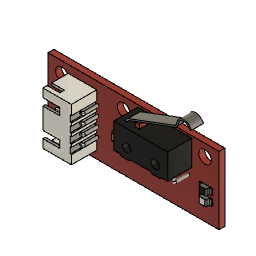
MetalFunk (Autodesk Fusion 360 archive; units mm, degrees)
design "End Stop Switch v5"
Autodesk Fusion 360 part; units mm, degrees
note: some values were not read from the file. Set by a fixed rule: which face or edge a step refers to.
sketch "Sketch1" plane through (0, 0, 0) normal (0, 1, 0) x (1, 0, 0)
  line L0 (20.25, 8.025) -> (-20.25, 8.025)
  line L1 (-20.25, 8.025) -> (-20.25, -8.025)
  line L2 (-20.25, -8.025) -> (20.25, -8.025)
  line L3 (20.25, -8.025) -> (20.25, 8.025)
  line L4 (20.25, 8.025) -> (-20.25, -8.025) construction
  line L5 (-20.25, 8.025) -> (20.25, -8.025) construction
  circle A0 centre (-16.95, -5.25) radius 1.5
  circle A1 centre (-16.95, 5.25) radius 1.5
  line L6 (-16.95, 5.25) -> (-16.95, -5.25) construction
  line L7 (-20.25, 0) -> (-16.95, 0) construction
  circle A2 centre (16.95, -5.25) radius 1.5
  line L8 (-16.95, -5.25) -> (16.95, -5.25) construction
  circle A3 centre (-2.35, -5.25) radius 1.5
  dimension "d1" = 40.5
  dimension "d2" = 16.05
  dimension "d3" = 3
  dimension "d4" = 10.5
  dimension "d5" = 3.3
  dimension "d6" = 3.3
  dimension "d7" = 3
  dimension "d8" = 14.6
  constraint horizontal L0
  constraint perpendicular L0 L1
  constraint parallel L0 L2
  constraint parallel L1 L3
  constraint coincident L4 origin
  constraint coincident L5 origin
  constraint equal A0 A1
  constraint coincident A1.centre L6.start
  constraint coincident A0.centre L6.end
  constraint vertical L6
  constraint midpoint L1 L7.start
  constraint midpoint L6 L7.end
  constraint horizontal L7
  constraint equal A0 A2
  constraint coincident A2.centre L8.end
  constraint horizontal L8
  constraint coincident L8 A3.centre
  measures "d1" distance of L0.start L0.end
  measures "d2" distance of L0.start L2.end
  measures "d3" diameter of A0
  measures "d4" distance of A0.centre A1.centre
  measures "d5" distance of L1 A0.centre
  measures "d6" distance of L3 A2.centre
  measures "d7" diameter of A3
  measures "d8" distance of A0.centre A3.centre
extrude "Extrude1" add sketch "Sketch1" along normal blind 1.4
sketch "Sketch2" plane through (0, 1.4, 0) normal (0, 1, 0) x (-1, 0, 0)
  circle A0 centre (2.35, 5.25) radius 1.5
  circle A1 centre (-16.95, 5.25) radius 1.5
  circle A2 centre (16.95, -5.25) radius 1.5
  circle A3 centre (16.95, 5.25) radius 1.5
  line L0 (-20.25, 8.025) -> (-20.25, -8.025)
  line L1 (-20.25, -8.025) -> (20.25, -8.025)
  line L2 (20.25, -8.025) -> (20.25, 8.025)
  line L3 (20.25, 8.025) -> (-20.25, 8.025)
  line L4 (7.75, 2.225) -> (9.25, 2.225)
  arc A4 (9.25, 2.225) -> (9.25, 4.025) centre (9.25, 3.125) ccw
  line L5 (9.25, 4.025) -> (7.75, 4.025)
  arc A5 (7.75, 4.025) -> (7.75, 2.225) centre (7.75, 3.125) ccw
  line L6 (7.75, 3.125) -> (9.25, 3.125) construction
  line L7 (9.25, 1.8583) -> (7.75, 1.8583)
  arc A6 (7.75, 1.8583) -> (7.75, 0.0583) centre (7.75, 0.9583) ccw
  line L8 (7.75, 0.0583) -> (9.25, 0.0583)
  arc A7 (9.25, 0.0583) -> (9.25, 1.8583) centre (9.25, 0.9583) ccw
  line L9 (9.25, -0.3083) -> (7.75, -0.3083)
  arc A8 (7.75, -0.3083) -> (7.75, -2.1083) centre (7.75, -1.2083) ccw
  line L10 (7.75, -2.1083) -> (9.25, -2.1083)
  arc A9 (9.25, -2.1083) -> (9.25, -0.3083) centre (9.25, -1.2083) ccw
  line L11 (9.25, -2.475) -> (7.75, -2.475)
  arc A10 (7.75, -2.475) -> (7.75, -4.275) centre (7.75, -3.375) ccw
  line L12 (7.75, -4.275) -> (9.25, -4.275)
  arc A11 (9.25, -4.275) -> (9.25, -2.475) centre (9.25, -3.375) ccw
  circle A12 centre (8.5, 3.125) radius 0.3
  circle A13 centre (8.5, 0.9583) radius 0.3
  circle A14 centre (8.5, -1.2083) radius 0.3
  circle A15 centre (8.5, -3.375) radius 0.3
  line L13 (-13.95, 0.475) -> (-13.95, -1.025)
  arc A16 (-13.95, -1.025) -> (-12.15, -1.025) centre (-13.05, -1.025) ccw
  line L14 (-12.15, -1.025) -> (-12.15, 0.475)
  arc A17 (-12.15, 0.475) -> (-13.95, 0.475) centre (-13.05, 0.475) ccw
  line L15 (-13.05, 0.475) -> (-13.05, -1.025) construction
  line L16 (-6.65, -1.025) -> (-6.65, 0.475)
  arc A18 (-6.65, 0.475) -> (-8.45, 0.475) centre (-7.55, 0.475) ccw
  line L17 (-8.45, 0.475) -> (-8.45, -1.025)
  arc A19 (-8.45, -1.025) -> (-6.65, -1.025) centre (-7.55, -1.025) ccw
  line L18 (-1.15, -1.025) -> (-1.15, 0.475)
  arc A20 (-1.15, 0.475) -> (-2.95, 0.475) centre (-2.05, 0.475) ccw
  line L19 (-2.95, 0.475) -> (-2.95, -1.025)
  arc A21 (-2.95, -1.025) -> (-1.15, -1.025) centre (-2.05, -1.025) ccw
  circle A22 centre (-13.05, -0.275) radius 0.3
  line L20 (-7.55, 0.475) -> (-7.55, -1.025) construction
  line L21 (-2.05, -1.025) -> (-2.05, 0.475) construction
  circle A23 centre (-7.55, -0.275) radius 0.3
  circle A24 centre (-2.05, -0.275) radius 0.3
  dimension "d11" = 1.8
  dimension "d12" = 1.5
  dimension "d13" = 4
  dimension "d14" = 11
  dimension "d17" = 0
  dimension "d18" = -6.5
  dimension "d19" = 0.6
  dimension "d30" = 1.5
  dimension "d31" = 1.8
  dimension "d32" = 7
  dimension "d33" = 7.2
  dimension "d36" = 11
  dimension "d37" = 0
  dimension "d38" = 0.6
  constraint tangent L4 A4
  constraint tangent A4 L5
  constraint parallel L4 L5
  constraint tangent L5 A5
  constraint tangent L4 A5
  constraint horizontal L6
  constraint midpoint L6 A12.centre
  constraint equal A14 A15
  constraint equal A13 A14
  constraint equal A12 A13
  constraint tangent L13 A16
  constraint tangent A16 L14
  constraint parallel L13 L14
  constraint tangent L14 A17
  constraint tangent L13 A17
  constraint parallel L0 L15
  constraint midpoint L15 A22.centre
  constraint coincident A18.centre L20.start
  constraint coincident A19.centre L20.end
  constraint coincident A21.centre L21.start
  constraint coincident A20.centre L21.end
  constraint midpoint L20 A23.centre
  constraint midpoint L21 A24.centre
  constraint equal A22 A23
  constraint equal A23 A24
  measures "d11" distance of L4 L5
  measures "d12" distance of A5.centre A4.centre
  measures "d13" distance of L3 L5
  measures "d14" distance of L2 A4.centre
  measures "d19" diameter of A15
  measures "d30" distance of A17.centre A16.centre
  measures "d31" distance of L13 L14
  measures "d32" distance of L1 A16.centre
  measures "d33" distance of L0 A16.centre
  measures "d38" diameter of A22
extrude "Extrude6" add sketch "Sketch2" against normal blind 4.35 contours A12 | A13 | A14 | A15
extrude "Extrude2" add sketch "Sketch2" along normal blind 0.5 contours L4 A4 L5 A5 | L7 A6 L8 A7 | L9 A8 L10 A9 | L11 A10 L12 A11 | L13 A16 L14 A17 | L16 A18 L17 A19 | L18 A20 L19 A21
extrude "Extrude3" add sketch "Sketch2" along normal blind 2 contours A12 | A13 | A14 | A15 | A22 | A23 | A24
fillet "Fillet1" radius 0.3 1 faces at (-8.4925, 1.9, -4.0747)
fillet "Fillet2" radius 0.3 3 faces at (-8.4925, 1.9, -1.9081) (-8.4925, 1.9, 0.2586) (-8.4925, 1.9, 2.4253)
fillet "Fillet2" radius 0.3 3 faces at (13.75, 1.9, -0.275) (6.85, 1.9, -0.275) (2.75, 1.9, -0.275)
fillet "Fillet3" radius 0.1 1 edges at (-8.2203, 3.4, 3.0165) 4 faces at (-8.4377, 3.4, -3.5121) (-8.4377, 3.4, -1.3455) (-8.4267, 3.4, 0.8314) (-8.4377, 3.4, 2.9879)
fillet "Fillet3" radius 0.1 3 faces at (2.1033, 3.4, -0.0705) (7.6233, 3.4, -0.148) (12.9767, 3.4, -0.148)
sketch "Sketch3" plane through (0, 0, 0) normal (0, -1, 0) x (1, 0, 0)
  circle A0 centre (-2.35, 5.25) radius 1.5
  circle A1 centre (16.95, 5.25) radius 1.5
  circle A2 centre (-16.95, -5.25) radius 1.5
  circle A3 centre (-16.95, 5.25) radius 1.5
  line L0 (20.25, -8.025) -> (20.25, 8.025)
  line L1 (20.25, 8.025) -> (-20.25, 8.025)
  line L2 (-20.25, 8.025) -> (-20.25, -8.025)
  line L3 (-20.25, -8.025) -> (20.25, -8.025)
  line L4 (-15.45, 6.2) -> (-8.7, 6.2)
  line L5 (-8.7, 6.2) -> (-8.7, -6.2)
  line L6 (-8.7, -6.2) -> (-15.45, -6.2)
  line L7 (-15.45, -6.2) -> (-15.45, 6.2)
  line L8 (-20.25, 0) -> (-15.45, 0) construction
  circle A4 centre (-8.5, -3.375) radius 0.3
  circle A5 centre (-8.5, 0.9583) radius 0.3
  circle A6 centre (-8.5, -1.2083) radius 0.3
  circle A7 centre (-8.5, 3.125) radius 0.3
  dimension "d43" = 12.4
  dimension "d44" = 6.75
  constraint horizontal L4
  constraint vertical L5
  constraint horizontal L6
  constraint vertical L7
  constraint tangent A3 L7
  constraint midpoint L2 L8.start
  constraint midpoint L7 L8.end
  constraint horizontal L8
  measures "d43" distance of L4 L6
  measures "d44" distance of L4.start L4.end
extrude "Extrude4" add sketch "Sketch3" along normal blind 6 contours L4 L5 L6 L7 A4 A5 A6 A7 | L5 A4 | L5 A7 | L5 A6 | L5 A5 picked at (-8.7489, -3.4027) picked at (-8.7504, 3.1324) picked at (-8.718, -1.2615) picked at (-8.7504, 0.9657)
sketch "Sketch4" plane through (-15.45, 0, 0) normal (-1, 0, 0) x (0, -1, 0)
  line L0 (0, -5.25) -> (0, -6.2)
  line L1 (0, -6.2) -> (6, -6.2)
  line L2 (6, -6.2) -> (6, 6.2)
  line L3 (6, 6.2) -> (0, 6.2)
  line L4 (0, 6.2) -> (0, 5.25)
  line L5 (0, 5.25) -> (0, -5.25)
  line L6 (0.6, 5.6) -> (0.6, 5.25)
  line L7 (0.6, 5.25) -> (0.6, -5.25)
  line L8 (0.6, -5.25) -> (0.6, -5.6)
  line L9 (0.6, -5.6) -> (5.4, -5.6)
  line L10 (5.4, -5.6) -> (5.4, 5.6)
  line L11 (5.4, 5.6) -> (0.6, 5.6)
  dimension "d47" = -0.6
extrude "Extrude5" cut sketch "Sketch4" against normal blind 6.15 contours L6 L7 L8 L9 L10 L11
ref_plane "WorkPlane1" through (-12.075, -3, 3.2) normal (0, 0, 1) x (-1, 0, 0)
sketch "Sketch6" plane through (0, -6, 0) normal (0, -1, 0) x (1, 0, 0)
  line L0 (-15.45, -6.2) -> (-8.7, -6.2)
  line L1 (-8.7, 1.7083) -> (-8.7, 2.375)
  line L2 (-8.7, 6.2) -> (-15.45, 6.2)
  line L3 (-15.45, 6.2) -> (-15.45, -6.2)
  line L4 (-15.45, 4.2) -> (-11.45, 4.2)
  line L5 (-11.45, 4.2) -> (-11.45, 2.5)
  line L6 (-11.45, 2.5) -> (-15.45, 2.5)
  line L7 (-15.45, 2.5) -> (-15.45, 4.2)
  line L8 (-15.45, -2.5) -> (-11.45, -2.5)
  line L9 (-11.45, -2.5) -> (-11.45, -4.2)
  line L10 (-11.45, -4.2) -> (-15.45, -4.2)
  line L11 (-15.45, -4.2) -> (-15.45, -2.5)
  line L12 (-9, 1.7083) -> (-8.7, 1.7083)
  line L13 (-8.7, 2.375) -> (-9, 2.375)
  line L14 (-9, 2.375) -> (-9, 3.875)
  line L15 (-9, 3.875) -> (-8.7, 3.875)
  line L16 (-8.7, 3.875) -> (-8.7, 6.2)
  line L17 (-8.7, -6.2) -> (-8.7, -4.125)
  line L18 (-8.7, -4.125) -> (-9, -4.125)
  line L19 (-9, -4.125) -> (-9, -2.625)
  line L20 (-9, -2.625) -> (-8.7, -2.625)
  line L21 (-8.7, -2.625) -> (-8.7, -1.9583)
  line L22 (-8.7, -1.9583) -> (-9, -1.9583)
  line L23 (-9, -1.9583) -> (-9, -0.4583)
  line L24 (-9, -0.4583) -> (-8.7, -0.4583)
  line L25 (-8.7, -0.4583) -> (-8.7, 0.2083)
  line L26 (-8.7, 0.2083) -> (-9, 0.2083)
  line L27 (-9, 0.2083) -> (-9, 1.7083)
  dimension "d62" = 1.7
  dimension "d63" = 1.7
  dimension "d64" = 4
  dimension "d65" = 4
  dimension "d66" = 2
  dimension "d67" = 2
  constraint horizontal L4
  constraint vertical L5
  constraint horizontal L6
  constraint vertical L7
  constraint coincident L3 L4.start
  constraint horizontal L8
  constraint vertical L9
  constraint horizontal L10
  constraint vertical L11
  constraint coincident L3 L8.start
  measures "d62" distance of L4 L6
  measures "d63" distance of L8 L10
  measures "d64" distance of L5.end L6.end
  measures "d65" distance of L9.end L10.end
  measures "d66" distance of L2 L4
  measures "d67" distance of L0 L10
extrude "Extrude8" cut sketch "Sketch6" against normal blind 1 contours L3 L8 L9 L10 L11 | L3 L4 L5 L6 L7
sketch "Sketch5" plane through (-12.075, -3, 3.2) normal (0, 0, 1) x (1, 0, 0)
  line L0 (3.6, 0.05) -> (3.6, -0.2)
  line L1 (3.3, -0.5) -> (2.75, -0.5)
  arc A0 (3.3, -0.5) -> (3.6, -0.2) centre (3.3, -0.2) ccw
  dimension "d53" = 0.3
  constraint vertical L0
  constraint perpendicular L0 L1
  constraint tangent L1 A0
  constraint tangent L0 A0
  measures "d53" radius of A0
sweep "Sweep1" add 4 faces at (-8.5336, -2.95, 3.1176) (-8.5336, -2.95, 0.9509) (-8.5336, -2.95, -1.2157) (-8.5336, -2.95, -3.3824) path "Sketch5" along L1 A0 L0
sketch "Sketch7" plane through (0, -6, 0) normal (0, -1, 0) x (1, 0, 0)
  line L0 (-11.45, 2.5) -> (-15.45, 2.5)
  line L1 (-15.45, 2.5) -> (-15.45, -2.5)
  line L2 (-15.45, -2.5) -> (-11.45, -2.5)
  line L3 (-11.45, -2.5) -> (-11.45, -4.2)
  line L4 (-11.45, -4.2) -> (-15.45, -4.2)
  line L5 (-15.45, -4.2) -> (-15.45, -6.2)
  line L6 (-15.45, -6.2) -> (-8.7, -6.2)
  line L7 (-8.7, -6.2) -> (-8.7, 6.2)
  line L8 (-8.7, 6.2) -> (-15.45, 6.2)
  line L9 (-15.45, 6.2) -> (-15.45, 4.2)
  line L10 (-15.45, 4.2) -> (-11.45, 4.2)
  line L11 (-11.45, 4.2) -> (-11.45, 2.5)
  line L12 (-8.7, 3.875) -> (-9, 3.875)
  line L13 (-9, 3.875) -> (-9, 2.375)
  line L14 (-9, 2.375) -> (-8.7, 2.375)
  line L15 (-8.7, 2.375) -> (-8.7, 3.875)
  arc A0 (-8.7, 2.9014) -> (-8.7, 3.3486) centre (-8.5, 3.125) ccw construction
  line L16 (-9, 3.125) -> (-8.5, 3.125) construction
  line L17 (-8.7, 1.7083) -> (-9, 1.7083)
  line L18 (-8.7, 0.2083) -> (-8.7, 1.7083)
  line L19 (-9, 1.7083) -> (-9, 0.2083)
  line L20 (-9, 0.2083) -> (-8.7, 0.2083)
  line L21 (-8.7, -0.4583) -> (-9, -0.4583)
  line L22 (-8.7, -1.9583) -> (-8.7, -0.4583)
  line L23 (-9, -0.4583) -> (-9, -1.9583)
  line L24 (-9, -1.9583) -> (-8.7, -1.9583)
  line L25 (-8.7, -2.625) -> (-9, -2.625)
  line L26 (-8.7, -4.125) -> (-8.7, -2.625)
  line L27 (-9, -2.625) -> (-9, -4.125)
  line L28 (-9, -4.125) -> (-8.7, -4.125)
  dimension "d70" = 0.3
  dimension "d71" = 1.5
  dimension "d74" = 0
  dimension "d75" = -6.5
  constraint horizontal L12
  constraint vertical L13
  constraint horizontal L14
  constraint vertical L15
  constraint coincident L7 L12.start
  constraint midpoint L13 L16.start
  constraint coincident A0.centre L16.end
  constraint horizontal L16
  measures "d70" distance of L13.end L14.end
  measures "d71" distance of L12.end L13.end
extrude "Extrude9" cut sketch "Sketch7" against normal blind 6 contours L7 L12 L13 L14 L15 | L7 L17 L18 L19 L20 | L7 L25 L26 L27 L28 | L7 L21 L22 L23 L24
extrude "Extrude7" add 4 faces at (-9.325, -3.4102, 3.0521) (-9.325, -3.4102, 0.8855) (-9.325, -3.4102, -1.2812) (-9.325, -3.4102, -3.4479) along direction (-1, 0, 0) blind 5.5 and the other way blind 0.63
sketch "Sketch8" plane through (0, 0, -6.2) normal (0, 0, -1) x (1, 0, 0)
  line L0 (-15.45, 0) -> (-8.7, 0)
  line L1 (-8.7, 0) -> (-8.7, 6)
  line L2 (-8.7, 6) -> (-15.45, 6)
  line L3 (-15.45, 6) -> (-15.45, 0)
  line L4 (-15.45, 5) -> (-12.45, 5)
  line L5 (-12.45, 5) -> (-12.45, 3.9)
  line L6 (-12.45, 3.9) -> (-15.45, 3.9)
  line L7 (-15.45, 3.9) -> (-15.45, 5)
  dimension "d80" = 1.1
  dimension "d81" = 1
  dimension "d82" = 3
  constraint horizontal L4
  constraint vertical L5
  constraint horizontal L6
  constraint vertical L7
  constraint coincident L3 L4.start
  measures "d80" distance of L4.end L5.end
  measures "d81" distance of L2 L4
  measures "d82" distance of L5.end L6.end
extrude "Extrude10" cut sketch "Sketch8" against normal blind 1 contours L3 L4 L5 L6 L7
mirror "Mirror1" about plane through (0, 0, 0) normal (0, 0, 1) of "Extrude10"
sketch "Sketch9" plane through (0, 0, 0) normal (0, -1, 0) x (1, 0, 0)
  arc A0 (-8.7, 0.7347) -> (-8.7, 1.1819) centre (-8.5, 0.9583) ccw
  line L0 (-8.7, 0.7347) -> (-8.7, 1.1819)
  arc A1 (-8.7, -1.4319) -> (-8.7, -0.9847) centre (-8.5, -1.2083) ccw
  line L1 (-8.7, -1.4319) -> (-8.7, -0.9847)
  arc A2 (-8.7, 2.9014) -> (-8.7, 3.3486) centre (-8.5, 3.125) ccw
  line L2 (-8.7, 2.9014) -> (-8.7, 3.3486)
  line L3 (-8.7, 1.7083) -> (-9, 1.7083)
  line L4 (-9, 1.7083) -> (-9, 0.2083)
  line L5 (-9, 0.2083) -> (-8.7, 0.2083)
  line L6 (-8.7, 0.2083) -> (-8.7, -0.4583)
  line L7 (-8.7, -0.4583) -> (-9, -0.4583)
  line L8 (-9, -0.4583) -> (-9, -1.9583)
  line L9 (-9, -1.9583) -> (-8.7, -1.9583)
  line L10 (-8.7, -1.9583) -> (-8.7, -2.625)
  line L11 (-8.7, -2.625) -> (-9, -2.625)
  line L12 (-9, -2.625) -> (-9, -4.125)
  line L13 (-9, -4.125) -> (-8.7, -4.125)
  line L14 (-8.7, -4.125) -> (-8.7, -6.2)
  line L15 (-8.7, -6.2) -> (-15.45, -6.2)
  line L16 (-15.45, -6.2) -> (-15.45, -5.25)
  circle A3 centre (-16.95, -5.25) radius 1.5
  line L17 (-15.45, -5.25) -> (-15.45, 5.25)
  circle A4 centre (-16.95, 5.25) radius 1.5
  line L18 (-15.45, 5.25) -> (-15.45, 6.2)
  line L19 (-15.45, 6.2) -> (-8.7, 6.2)
  line L20 (-8.7, 6.2) -> (-8.7, 3.875)
  line L21 (-8.7, 3.875) -> (-9, 3.875)
  line L22 (-9, 3.875) -> (-9, 2.375)
  line L23 (-9, 2.375) -> (-8.7, 2.375)
  line L24 (-8.7, 2.375) -> (-8.7, 1.7083)
  line L25 (20.25, -8.025) -> (20.25, 8.025)
  line L26 (20.25, 8.025) -> (-20.25, 8.025)
  line L27 (-20.25, 8.025) -> (-20.25, -8.025)
  line L28 (-20.25, -8.025) -> (20.25, -8.025)
  circle A5 centre (16.95, 5.25) radius 1.5
  circle A6 centre (-2.35, 5.25) radius 1.5
  line L29 (-8.7, -3.5986) -> (-8.7, -3.1514)
  arc A7 (-8.7, -3.5986) -> (-8.7, -3.1514) centre (-8.5, -3.375) ccw
  line L30 (-4.15, 0.475) -> (-2.75, 0.475)
  line L31 (-2.75, 0.475) -> (-2.75, -1.725)
  line L32 (-2.75, -1.725) -> (-4.15, -1.725)
  line L33 (-4.15, -1.725) -> (-4.15, 0.475)
  line L34 (-4.15, 0.875) -> (-2.75, 0.875)
  line L35 (-2.75, 0.875) -> (-2.75, -2.125)
  line L36 (-2.75, -2.125) -> (-4.15, -2.125)
  line L37 (-4.15, -2.125) -> (-4.15, 0.875)
  line L38 (-4.15, -0.625) -> (-2.75, -0.625) construction
  line L39 (-0.05, 0.875) -> (-0.0503, 0.8857)
  line L40 (-1.95, 0.8566) -> (-1.95, 0.875)
  line L41 (-1.95, 0.875) -> (-0.55, 0.875)
  line L42 (-0.55, 0.875) -> (-0.55, -2.125)
  line L43 (-0.55, -2.125) -> (-1.95, -2.125)
  line L44 (-1.95, -2.125) -> (-1.95, 0.875)
  line L45 (-1.95, 0.475) -> (-0.55, 0.475)
  line L46 (-0.55, 0.475) -> (-0.55, -1.725)
  line L47 (-0.55, -1.725) -> (-1.95, -1.725)
  line L48 (-1.95, -1.725) -> (-1.95, 0.475)
  dimension "d87" = 2.2
  dimension "d88" = 1.4
  dimension "d89" = 8.5
  dimension "d90" = 17.5
  dimension "d91" = 3
  dimension "d97" = 0.8
  constraint horizontal L30
  constraint vertical L31
  constraint horizontal L32
  constraint vertical L33
  constraint horizontal L34
  constraint vertical L35
  constraint horizontal L36
  constraint vertical L37
  constraint collinear L33 L37
  constraint collinear L31 L35
  constraint midpoint L37 L38.start
  constraint midpoint L35 L38.end
  constraint symmetric L30 L32 L38
  constraint horizontal L41
  constraint vertical L42
  constraint horizontal L43
  constraint vertical L44
  constraint equal L36 L43
  constraint equal L37 L44
  constraint horizontal L45
  constraint vertical L46
  constraint horizontal L47
  constraint vertical L48
  constraint coincident L42 L46.end
  constraint coincident L44 L45.start
  constraint collinear L32 L47
  constraint collinear L30 L45
  constraint collinear L34 L41
  measures "d87" distance of L30.end L31.end
  measures "d88" distance of L31.end L32.end
  measures "d89" distance of L28 L30
  measures "d90" distance of L27 L31
  measures "d91" distance of L34 L36
  measures "d97" distance of L35 L40
extrude "Extrude11" add sketch "Sketch9" along normal blind 0.2 contours L30 L34 L35 L37 | L32 L35 L36 L37 | L40 L41 L42 L44 L45 | L42 L43 L44 L47
extrude "Extrude12" add sketch "Sketch9" along normal blind 1 contours L30 L31 L32 L33 L35 L37 | L42 L44 L45 L46 L47 L48
fillet "Fillet4" radius 0.4 4 edges at (-3.45, -1, -1.725) (-3.45, -1, 0.475) (-1.25, -1, 0.475) (-1.25, -1, -1.725)
sketch "Sketch10" plane through (0, 0, 0) normal (0, -1, 0) x (1, 0, 0)
  line L0 (-0.55, 0.875) -> (-0.55, -2.125)
  line L1 (-0.55, -2.125) -> (-1.95, -2.125)
  line L2 (-1.95, -2.125) -> (-1.95, 0.875)
  line L3 (-1.95, 0.875) -> (-0.55, 0.875)
  line L4 (-8.7, -3.5986) -> (-8.7, -3.1514)
  arc A0 (-8.7, -3.5986) -> (-8.7, -3.1514) centre (-8.5, -3.375) ccw
  circle A1 centre (-2.35, 5.25) radius 1.5
  circle A2 centre (16.95, 5.25) radius 1.5
  line L5 (20.25, -8.025) -> (20.25, 8.025)
  line L6 (20.25, 8.025) -> (-20.25, 8.025)
  line L7 (-20.25, 8.025) -> (-20.25, -8.025)
  line L8 (-20.25, -8.025) -> (20.25, -8.025)
  line L9 (-8.7, 1.7083) -> (-9, 1.7083)
  line L10 (-9, 1.7083) -> (-9, 0.2083)
  line L11 (-9, 0.2083) -> (-8.7, 0.2083)
  line L12 (-8.7, 0.2083) -> (-8.7, -0.4583)
  line L13 (-8.7, -0.4583) -> (-9, -0.4583)
  line L14 (-9, -0.4583) -> (-9, -1.9583)
  line L15 (-9, -1.9583) -> (-8.7, -1.9583)
  line L16 (-8.7, -1.9583) -> (-8.7, -2.625)
  line L17 (-8.7, -2.625) -> (-9, -2.625)
  line L18 (-9, -2.625) -> (-9, -4.125)
  line L19 (-9, -4.125) -> (-8.7, -4.125)
  line L20 (-8.7, -4.125) -> (-8.7, -6.2)
  line L21 (-8.7, -6.2) -> (-15.45, -6.2)
  line L22 (-15.45, -6.2) -> (-15.45, -5.25)
  circle A3 centre (-16.95, -5.25) radius 1.5
  line L23 (-15.45, -5.25) -> (-15.45, 5.25)
  circle A4 centre (-16.95, 5.25) radius 1.5
  line L24 (-15.45, 5.25) -> (-15.45, 6.2)
  line L25 (-15.45, 6.2) -> (-8.7, 6.2)
  line L26 (-8.7, 6.2) -> (-8.7, 3.875)
  line L27 (-8.7, 3.875) -> (-9, 3.875)
  line L28 (-9, 3.875) -> (-9, 2.375)
  line L29 (-9, 2.375) -> (-8.7, 2.375)
  line L30 (-8.7, 2.375) -> (-8.7, 1.7083)
  arc A5 (-8.7, 2.9014) -> (-8.7, 3.3486) centre (-8.5, 3.125) ccw
  line L31 (-8.7, 2.9014) -> (-8.7, 3.3486)
  arc A6 (-8.7, -1.4319) -> (-8.7, -0.9847) centre (-8.5, -1.2083) ccw
  line L32 (-8.7, -1.4319) -> (-8.7, -0.9847)
  arc A7 (-8.7, 0.7347) -> (-8.7, 1.1819) centre (-8.5, 0.9583) ccw
  line L33 (-8.7, 0.7347) -> (-8.7, 1.1819)
  line L34 (-4.15, -2.125) -> (-4.15, 0.875)
  line L35 (-4.15, 0.875) -> (-2.75, 0.875)
  line L36 (-2.75, 0.875) -> (-2.75, -2.125)
  line L37 (-2.75, -2.125) -> (-4.15, -2.125)
  line L38 (1.05, 7.525) -> (13.8, 7.525)
  line L39 (13.8, 7.525) -> (13.8, 1.525)
  line L40 (1.05, 1.525) -> (1.05, 7.525)
  circle A8 centre (4.05, 3.525) radius 1
  circle A9 centre (10.8, 3.525) radius 1
  line L41 (2.55, 1.475) -> (2.55, 1.525)
  line L42 (5.05, 1.475) -> (5.05, 1.525)
  line L43 (9.8, 1.475) -> (9.8, 1.525)
  line L44 (12.3, 1.475) -> (12.3, 1.525)
  line L45 (12, 1.175) -> (10.1, 1.175)
  line L46 (4.75, 1.175) -> (2.85, 1.175)
  line L47 (2.55, 1.525) -> (1.05, 1.525)
  line L48 (13.8, 1.525) -> (12.3, 1.525)
  line L49 (9.8, 1.525) -> (5.05, 1.525)
  line L50 (2.55, 1.475) -> (2.85, 1.175)
  line L51 (4.75, 1.175) -> (5.05, 1.475)
  line L52 (12.3, 1.475) -> (12, 1.175)
  line L53 (9.8, 1.475) -> (10.1, 1.175)
  point P0 (2.55, 1.175)
  point P1 (5.05, 1.175)
  point P2 (9.8, 1.175)
  point P3 (12.3, 1.175)
  dimension "d104" = 12.75
  dimension "d105" = 6
  dimension "d106" = 0.5
  dimension "d107" = 19.2
  dimension "d108" = 2
  dimension "d109" = 3
  dimension "d110" = 3
  dimension "d111" = 4
  dimension "d112" = 4
  dimension "d114" = 2.5
  dimension "d115" = 2.5
  dimension "d116" = 0.3
  dimension "d117" = 0.3
  dimension "d118" = 0.3
  dimension "d119" = 0.3
  dimension "d120" = 0.3
  dimension "d121" = 0.3
  dimension "d122" = 0.3
  dimension "d123" = 0.3
  dimension "d124" = 4
  dimension "d125" = 4
  constraint horizontal L38
  constraint vertical L39
  constraint horizontal L48
  constraint vertical L40
  constraint equal A8 A9
  constraint coincident L41.end L48
  constraint perpendicular L41 L48
  constraint coincident P1 L45
  constraint perpendicular L42 L48
  constraint coincident L43.end L48
  constraint perpendicular L43 L45
  constraint perpendicular L44 L48
  constraint parallel L45 L48
  constraint collinear L45 L46
  constraint collinear L47 L48
  constraint collinear L48 L49
  constraint coincident P0 L41
  constraint coincident P0 L46
  constraint coincident P1 L42
  constraint coincident P3 L44
  constraint coincident P3 L45
  constraint coincident P2 L43
  constraint coincident P2 L45
  measures "d104" distance of L39.end L40.start
  measures "d105" distance of L38.end L39.end
  measures "d106" distance of L6 L38
  measures "d107" distance of L5 L40
  measures "d108" diameter of A8
  measures "d109" distance of L40 A8.centre
  measures "d110" distance of L39 A9.centre
  measures "d111" distance of L38 A9.centre
  measures "d112" distance of L38 A8.centre
  measures "d114" distance of P0 P1
  measures "d115" distance of P2 P3
  measures "d116" distance of P0 L41.start
  measures "d117" distance of P0 L46.end
  measures "d118" distance of P1 L46.start
  measures "d119" distance of P1 L42.start
  measures "d120" distance of P3 L44.start
  measures "d121" distance of P3 L45.start
  measures "d122" distance of P2 L43.start
  measures "d123" distance of P2 L45.end
  measures "d124" distance of L39 L43
  measures "d125" distance of L40 L42
extrude "Extrude13" add sketch "Sketch10" along normal blind 5.7 contours L38 L39 L40 L41 L42 L43 L44 L45 L46 L47 L48 L49 L50 L51 L52 L53
extrude "Extrude14" add sketch "Sketch2" against normal blind 4.3 contours A22 | A23 | A24
sketch "Sketch11" plane through (0, 0, 0) normal (1, 0, 0) x (0, 1, 0)
  line L0 (-2.8, -0.3) -> (-3.1, -0.3)
  line L1 (-3.6, 0.2) -> (-3.6, 2)
  arc A0 (-3.6, 0.2) -> (-3.1, -0.3) centre (-3.1, 0.2) ccw
  dimension "d130" = 0.5
  constraint horizontal L0
  constraint perpendicular L0 L1
  constraint tangent L1 A0
  constraint tangent L0 A0
  measures "d130" radius of A0
sweep "Sweep2" add 1 faces at (2.1033, -2.9, -0.0705) path "Sketch11" along L0 A0 L1
sweep "Sweep4" add 2 faces at (7.6233, -2.9, -0.148) (12.9767, -2.9, -0.148) path "Sketch11" along L0 A0 L1
sketch "Sketch12" plane through (0, 0, 7.525) normal (0, 0, 1) x (-1, 0, 0)
  line L0 (-13.8, 0) -> (-1.05, 0)
  line L1 (-1.05, 0) -> (-1.05, 5.7)
  line L2 (-1.05, 5.7) -> (-13.8, 5.7)
  line L3 (-13.8, 5.7) -> (-13.8, 0)
  line L4 (-4.75, 1.7) -> (-5.75, 1.7)
  line L5 (-5.75, 1.7) -> (-5.75, 4.35)
  line L6 (-5.75, 4.35) -> (-4.75, 4.35)
  line L7 (-4.75, 4.35) -> (-4.75, 1.7)
  dimension "d149" = 2.65
  dimension "d150" = 1
  dimension "d151" = 4.7
  dimension "d152" = 4
  constraint horizontal L4
  constraint vertical L5
  constraint horizontal L6
  constraint vertical L7
  measures "d149" distance of L4.start L6.end
  measures "d150" distance of L4.start L4.end
  measures "d151" distance of L1 L5
  measures "d152" distance of L2 L4
extrude "Extrude15" add sketch "Sketch12" along normal blind 1 contours L4 L5 L6 L7
sketch "Sketch13" plane through (0, 0, 7.525) normal (0, 0, 1) x (-1, 0, 0)
  line L0 (-4.75, 4.35) -> (-4.75, 1.7)
  line L1 (-4.75, 1.7) -> (-5.75, 1.7)
  line L2 (-5.75, 1.7) -> (-5.75, 4.35)
  line L3 (-5.75, 4.35) -> (-4.75, 4.35)
  line L4 (-13.8, 0) -> (-1.05, 0)
  line L5 (-1.05, 0) -> (-1.05, 5.7)
  line L6 (-1.05, 5.7) -> (-13.8, 5.7)
  line L7 (-13.8, 5.7) -> (-13.8, 0)
  line L8 (-2.25, 1.35) -> (-2.75, 1.35)
  line L9 (-2.75, 1.35) -> (-2.75, 4.35)
  line L10 (-2.75, 4.35) -> (-2.25, 4.35)
  line L11 (-2.25, 4.35) -> (-2.25, 1.35)
  line L12 (-4.75, 1.7) -> (-4.75, 4.35)
  line L13 (-2.25, 2.85) -> (-2.75, 2.85) construction
  line L14 (-1.05, 2.85) -> (-13.8, 2.85) construction
  dimension "d155" = 3
  dimension "d156" = 0.5
  dimension "d157" = 2
  constraint horizontal L8
  constraint vertical L9
  constraint horizontal L10
  constraint vertical L11
  constraint midpoint L11 L13.start
  constraint midpoint L9 L13.end
  constraint midpoint L5 L14.start
  constraint midpoint L7 L14.end
  constraint collinear L13 L14
  measures "d155" distance of L8.start L10.end
  measures "d156" distance of L8.start L8.end
  measures "d157" distance of L9 L12
extrude "Extrude16" cut sketch "Sketch13" against normal blind 0.5 contours L8 L9 L10 L11
sketch "Sketch14" plane through (0, -1.35, 0) normal (0, -1, 0) x (1, 0, 0)
  line L0 (2.75, 7.525) -> (2.25, 7.525)
  line L1 (2.25, 7.525) -> (2.25, 7.025)
  line L2 (2.25, 7.025) -> (2.75, 7.025)
  line L3 (2.75, 7.025) -> (2.75, 7.525)
  line L4 (2.5, 7.025) -> (2.5, 7.9081)
  line L5 (2.5, 7.9081) -> (14.0885, 12.2503)
  spline S0 degree 5 poles (14.533, 12.7043) (14.5695, 12.808) (14.6395, 13.0092) (14.7362, 13.2918) (14.8567, 13.6293) (15.0363, 13.9777) (15.2873, 14.2451) (15.6385, 14.4217) (16.0656, 14.5143) (16.529, 14.5026) (16.9976, 14.339) (17.3542, 14.0426) (17.6026, 13.7048) (17.7587, 13.4251) (17.8344, 13.2717) knots 0 0 0 0 0 0 0.1 0.2 0.3 0.4 0.5 0.6 0.7 0.8 0.9 1 1 1 1 1 1
  arc A0 (14.0885, 12.2503) -> (14.533, 12.7043) centre (13.8254, 12.9526) ccw
  line L6 (17.5473, 13.8538) -> (18.1214, 12.6895)
  line L7 (15.2858, 14.2509) -> (15.876, 14.4923)
  point P0 (14.5, 12.4045)
  point P1 (15.5809, 14.3716)
  dimension "d160" = 12
  dimension "d161" = 0.75
  constraint midpoint L2 L4.start
  constraint perpendicular L0 L4
  constraint coincident P0 L5
  constraint tangent L5 A0
  constraint tangent S0 A0
  constraint midpoint S0.end L6
  constraint midpoint P1 L7
  measures "d160" horizontal distance of L4.end P0
  measures "d161" radius of A0
sketch "Sketch15" plane through (0, 0, 7.025) normal (0, 0, 1) x (-1, 0, 0)
  line L0 (-2.25, 4.35) -> (-2.75, 4.35)
  line L1 (-2.75, 4.35) -> (-2.75, 1.35)
  line L2 (-2.75, 1.35) -> (-2.25, 1.35)
  line L3 (-2.25, 1.35) -> (-2.25, 4.35)
  line L4 (-2.6736, 4.2736) -> (-2.6736, 1.4264)
  line L5 (-2.6736, 1.4264) -> (-2.3264, 1.4264)
  line L6 (-2.3264, 1.4264) -> (-2.3264, 4.2736)
  line L7 (-2.3264, 4.2736) -> (-2.6736, 4.2736)
  dimension "d162" = -0.0764
sweep "Sweep5" add profiles "Sketch15" path "Sketch14" along L4 L5 A0 S0 section 1 contours L4 L5 L6 L7
fillet "Fillet5" radius 1 2 edges at (2.3264, -2.85, 8.0284) (2.6736, -2.85, 7.7878)
sketch "Sketch16" plane through (0, 0, 0) normal (0, -1, 0) x (1, 0, 0)
  circle A0 centre (13.05, -0.275) radius 0.3
  circle A1 centre (7.55, -0.275) radius 0.3
  circle A2 centre (2.05, -0.275) radius 0.3
  line L0 (9.8, 1.525) -> (5.05, 1.525)
  line L1 (5.05, 1.525) -> (5.05, 1.475)
  line L2 (5.05, 1.475) -> (4.75, 1.175)
  line L3 (4.75, 1.175) -> (2.85, 1.175)
  line L4 (2.85, 1.175) -> (2.55, 1.475)
  line L5 (2.55, 1.475) -> (2.55, 1.525)
  line L6 (2.55, 1.525) -> (1.05, 1.525)
  line L7 (1.05, 1.525) -> (1.05, 7.525)
  line L8 (1.05, 7.525) -> (13.8, 7.525)
  line L9 (13.8, 7.525) -> (13.8, 1.525)
  line L10 (13.8, 1.525) -> (12.3, 1.525)
  line L11 (12.3, 1.525) -> (12.3, 1.475)
  line L12 (12.3, 1.475) -> (12, 1.175)
  line L13 (12, 1.175) -> (10.1, 1.175)
  line L14 (10.1, 1.175) -> (9.8, 1.475)
  line L15 (9.8, 1.475) -> (9.8, 1.525)
  line L16 (-0.55, 0.875) -> (-0.55, -2.125)
  line L17 (-0.55, -2.125) -> (-1.95, -2.125)
  line L18 (-1.95, -2.125) -> (-1.95, 0.875)
  line L19 (-1.95, 0.875) -> (-0.55, 0.875)
  line L20 (-8.7, -3.5986) -> (-8.7, -3.1514)
  arc A3 (-8.7, -3.5986) -> (-8.7, -3.1514) centre (-8.5, -3.375) ccw
  circle A4 centre (-2.35, 5.25) radius 1.5
  circle A5 centre (16.95, 5.25) radius 1.5
  line L21 (20.25, -8.025) -> (20.25, 8.025)
  line L22 (20.25, 8.025) -> (-20.25, 8.025)
  line L23 (-20.25, 8.025) -> (-20.25, -8.025)
  line L24 (-20.25, -8.025) -> (20.25, -8.025)
  line L25 (-8.7, 1.7083) -> (-9, 1.7083)
  line L26 (-9, 1.7083) -> (-9, 0.2083)
  line L27 (-9, 0.2083) -> (-8.7, 0.2083)
  line L28 (-8.7, 0.2083) -> (-8.7, -0.4583)
  line L29 (-8.7, -0.4583) -> (-9, -0.4583)
  line L30 (-9, -0.4583) -> (-9, -1.9583)
  line L31 (-9, -1.9583) -> (-8.7, -1.9583)
  line L32 (-8.7, -1.9583) -> (-8.7, -2.625)
  line L33 (-8.7, -2.625) -> (-9, -2.625)
  line L34 (-9, -2.625) -> (-9, -4.125)
  line L35 (-9, -4.125) -> (-8.7, -4.125)
  line L36 (-8.7, -4.125) -> (-8.7, -6.2)
  line L37 (-8.7, -6.2) -> (-15.45, -6.2)
  line L38 (-15.45, -6.2) -> (-15.45, -5.25)
  circle A6 centre (-16.95, -5.25) radius 1.5
  line L39 (-15.45, -5.25) -> (-15.45, 5.25)
  circle A7 centre (-16.95, 5.25) radius 1.5
  line L40 (-15.45, 5.25) -> (-15.45, 6.2)
  line L41 (-15.45, 6.2) -> (-8.7, 6.2)
  line L42 (-8.7, 6.2) -> (-8.7, 3.875)
  line L43 (-8.7, 3.875) -> (-9, 3.875)
  line L44 (-9, 3.875) -> (-9, 2.375)
  line L45 (-9, 2.375) -> (-8.7, 2.375)
  line L46 (-8.7, 2.375) -> (-8.7, 1.7083)
  arc A8 (-8.7, 2.9014) -> (-8.7, 3.3486) centre (-8.5, 3.125) ccw
  line L47 (-8.7, 2.9014) -> (-8.7, 3.3486)
  arc A9 (-8.7, -1.4319) -> (-8.7, -0.9847) centre (-8.5, -1.2083) ccw
  line L48 (-8.7, -1.4319) -> (-8.7, -0.9847)
  arc A10 (-8.7, 0.7347) -> (-8.7, 1.1819) centre (-8.5, 0.9583) ccw
  line L49 (-8.7, 0.7347) -> (-8.7, 1.1819)
  line L50 (-4.15, -2.125) -> (-4.15, 0.875)
  line L51 (-4.15, 0.875) -> (-2.75, 0.875)
  line L52 (-2.75, 0.875) -> (-2.75, -2.125)
  line L53 (-2.75, -2.125) -> (-4.15, -2.125)
  line L54 (15.75, -2.525) -> (18.75, -2.525)
  line L55 (18.75, -2.525) -> (18.75, -3.925)
  line L56 (18.75, -3.925) -> (15.75, -3.925)
  line L57 (15.75, -3.925) -> (15.75, -2.525)
  line L58 (15.75, -0.325) -> (18.75, -0.325)
  line L59 (18.75, -0.325) -> (18.75, -1.725)
  line L60 (18.75, -1.725) -> (15.75, -1.725)
  line L61 (15.75, -1.725) -> (15.75, -0.325)
  line L62 (-0.55, 0.875) -> (-1.95, 0.875)
  line L63 (17.25, -0.325) -> (17.25, -3.925) construction
  line L64 (16.35, -0.325) -> (18.15, -0.325)
  line L65 (18.15, -0.325) -> (18.15, -1.725)
  line L66 (18.15, -1.725) -> (16.35, -1.725)
  line L67 (16.35, -1.725) -> (16.35, -0.325)
  line L68 (16.35, -2.525) -> (18.15, -2.525)
  line L69 (18.15, -2.525) -> (18.15, -3.925)
  line L70 (18.15, -3.925) -> (16.35, -3.925)
  line L71 (16.35, -3.925) -> (16.35, -2.525)
  dimension "d171" = 1.8
  dimension "d172" = 5.5
  dimension "d173" = 4.5
  dimension "d174" = 0.8
  constraint horizontal L54
  constraint vertical L55
  constraint horizontal L56
  constraint vertical L57
  constraint horizontal L58
  constraint vertical L59
  constraint horizontal L60
  constraint vertical L61
  constraint equal L55 L59
  constraint equal L54 L60
  constraint equal L59 L62
  constraint equal L16 L60
  constraint midpoint L58 L63.start
  constraint midpoint L56 L63.end
  constraint vertical L63
  constraint horizontal L64
  constraint vertical L65
  constraint horizontal L66
  constraint vertical L67
  constraint coincident L60 L65.end
  constraint coincident L58 L64.start
  constraint horizontal L68
  constraint vertical L69
  constraint horizontal L70
  constraint vertical L71
  constraint coincident L56 L69.end
  constraint coincident L54 L68.start
  constraint symmetric L63 L65 L67
  constraint symmetric L63 L69 L71
  constraint equal L66 L70
  measures "d171" distance of L65 L67
  measures "d172" distance of L24 L54
  measures "d173" distance of L21 L57
  measures "d174" distance of L54 L66
extrude "Extrude17" add sketch "Sketch16" along normal blind 0.2 contours L54 L56 L57 L71 | L54 L56 L68 L69 L70 L71 | L54 L55 L56 L69 | L58 L60 L61 L67 | L58 L60 L64 L65 L66 L67 | L58 L59 L60 L65
extrude "Extrude18" add sketch "Sketch16" along normal blind 1 contours L54 L56 L68 L69 L70 L71 | L58 L60 L64 L65 L66 L67
fillet "Fillet6" radius 0.25 4 edges at (16.35, -1, -1.025) (18.15, -1, -1.025) (18.15, -1, -3.225) (16.35, -1, -3.225)
equation "d117 = d116"
equation "d119 = d118"
equation "d121 = d120"
equation "d123 = d122"
